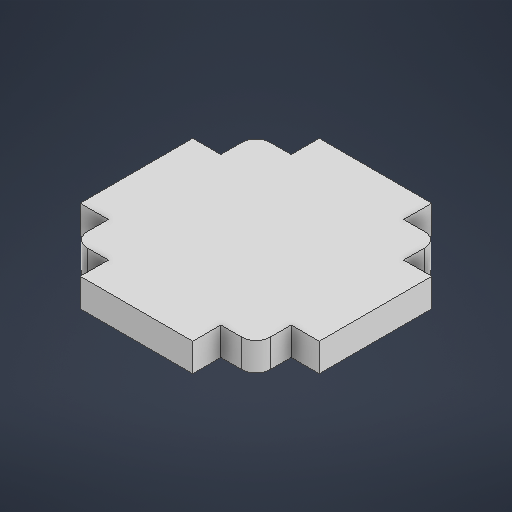
# Autodesk Inventor part: reference_magnet_lid
Saved by Autodesk Inventor 2026.1 (Build 301233020, 233B)
## iProperties
Created: 2025-11-29
Part Number: reference_magnet_lid
Material: Generic
Document SubType Name: Modeling
Designer: Carla Fernandez
Density: 1 g/cm^3
Appearance: Default
Author: Carla Fernandez
Autodesk Inventor part; units mm, degrees
ref_plane "YZ Plane" through (0, 0, 0) normal (1, 0, 0) x (0, 1, 0)
ref_plane "XZ Plane" through (0, 0, 0) normal (0, 1, 0) x (-1, 0, 0)
ref_plane "XY Plane" through (0, 0, 0) normal (0, 0, 1) x (1, 0, 0)
sketch "Sketch1" plane through (0, 0, 0) normal (0, 1, 0) x (-1, 0, 0)
  line L0 (7.2821, 0) -> (0, 0) construction
  line L1 (0, 0) -> (0, -6.7578) construction
  line L2 (8.5, 0) -> (8.5, -4)
  line L3 (8.5, -4) -> (6.5, -4)
  line L4 (4, -6.5) -> (4, -8.5)
  line L5 (4, -8.5) -> (0, -8.5)
  line L6 (6.5, -4) -> (6.5, -5.5)
  line L7 (5.5, -6.5) -> (4, -6.5)
  arc A0 (5.5, -6.5) -> (6.5, -5.5) centre (5.5, -5.5) ccw
  line L8 (-8.5, 0) -> (-8.5, -4)
  line L9 (-8.5, -4) -> (-6.5, -4)
  line L10 (-4, -6.5) -> (-4, -8.5)
  line L11 (-4, -8.5) -> (0, -8.5)
  line L12 (-6.5, -4) -> (-6.5, -5.5)
  line L13 (-5.5, -6.5) -> (-4, -6.5)
  arc A1 (-6.5, -5.5) -> (-5.5, -6.5) centre (-5.5, -5.5) ccw
  line L14 (0, 0) -> (0, 6.7578) construction
  line L15 (8.5, 0) -> (8.5, 4)
  line L16 (8.5, 4) -> (6.5, 4)
  line L17 (4, 6.5) -> (4, 8.5)
  line L18 (4, 8.5) -> (0, 8.5)
  line L19 (6.5, 4) -> (6.5, 5.5)
  line L20 (5.5, 6.5) -> (4, 6.5)
  arc A2 (6.5, 5.5) -> (5.5, 6.5) centre (5.5, 5.5) ccw
  line L21 (-8.5, 4) -> (-6.5, 4)
  line L22 (-4, 6.5) -> (-4, 8.5)
  line L23 (-6.5, 4) -> (-6.5, 5.5)
  line L24 (-5.5, 6.5) -> (-4, 6.5)
  arc A3 (-5.5, 6.5) -> (-6.5, 5.5) centre (-5.5, 5.5) ccw
  line L25 (-4, 8.5) -> (0, 8.5)
  line L26 (-8.5, 0) -> (-8.5, 4)
  point P0 (2, -8.5)
  point P1 (-2, -8.5)
  point P2 (2, 8.5)
  point P3 (-2, 8.5)
  dimension "d0" = 4
  dimension "d1" = 4
  dimension "d2" = 8.5
  dimension "d3" = 8.5
  dimension "d4" = 2
  dimension "d5" = 2
  dimension "d6" = 1
  constraints: 54 end point, 27 symmetric about line, 8 point on circle, 7 perpendicular, 4 centre point, 3 point on line, 2 tangent, 1 horizontal, 1 midpoint, 3 other
  measures "d0" distance between parallel lines of L3 L0
  measures "d1" distance between parallel lines of L1 L4
  measures "d2" distance between parallel lines of L2 L1
  measures "d3" distance between parallel lines of L5 L0
  measures "d4" distance between parallel lines of L6 L2
  measures "d5" distance from line of L7 point (2, -8.5)
  measures "d6" radius of A0
extrude "Extrusion1" add sketch "Sketch1" along normal blind 2
equation "\"d1\" = d0"
equation "\"d3\" = d2"
body "Solid1"
